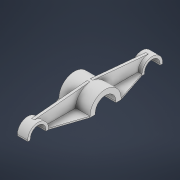
# Autodesk Inventor part: Pieza de practica 10
Saved by Autodesk Inventor 2022 (Build 260153000, 153)
## iProperties
Created: 2022-08-03
Part Number: Pieza de practica 10
Material: Genérico
Document SubType Name: Modeling
Designer: aleon
Density: 1 g/cm^3
Appearance: Valor por defecto
Author: aleon
Autodesk Inventor part; units mm, degrees
ref_plane "YZ Plane" through (0, 0, 0) normal (1, 0, 0) x (0, 1, 0)
ref_plane "XZ Plane" through (0, 0, 0) normal (0, 1, 0) x (-1, 0, 0)
ref_plane "XY Plane" through (0, 0, 0) normal (0, 0, 1) x (1, 0, 0)
sketch "Boceto1" plane through (0, 0, 0) normal (1, 0, 0) x (0, 1, 0)
  arc A0 (0, -20) -> (0, 20) centre (0, 0) ccw
  arc A1 (0, -30) -> (0, 30) centre (0, 0) ccw
  line L0 (0, 0) -> (-5, 0) construction
  arc A2 (0, -125) -> (0, -95) centre (0, -110) ccw
  arc A3 (0, -130) -> (0, -90) centre (0, -110) ccw
  arc A4 (0, 95) -> (0, 125) centre (0, 110) ccw
  arc A5 (0, 90) -> (0, 130) centre (0, 110) ccw
  line L1 (0, 95) -> (-2.5, 95)
  line L2 (-2.5, 95) -> (-2.5, 90)
  line L3 (-2.5, 90) -> (0, 90)
  line L4 (0, 125) -> (-2.5, 125)
  line L5 (-2.5, 125) -> (-2.5, 130)
  line L6 (-2.5, 130) -> (0, 130)
  line L7 (0, -95) -> (-2.5, -95)
  line L8 (-2.5, -95) -> (-2.5, -90)
  line L9 (-2.5, -90) -> (0, -90)
  line L10 (0, -125) -> (-2.5, -125)
  line L11 (-2.5, -125) -> (-2.5, -130)
  line L12 (-2.5, -130) -> (0, -130)
  line L13 (0, 20) -> (-2.5, 20)
  line L14 (-2.5, 20) -> (-2.5, 30)
  line L15 (-2.5, 30) -> (0, 30)
  line L16 (0, -20) -> (-2.5, -20)
  line L17 (-2.5, -20) -> (-2.5, -30)
  line L18 (-2.5, -30) -> (0, -30)
  point P0 (0, 130)
  dimension "d0" = 20
  dimension "d1" = 30
  dimension "d2" = 5
  dimension "d3" = 15
  dimension "d5" = 20
  dimension "d6" = 110
  dimension "d7" = 2.5
  dimension "d8" = 5
  dimension "d9" = 5
  dimension "d10" = 10
  dimension "d11" = 10
  dimension "d16" = 2.5
  constraints: 38 end point, 12 point on circle, 9 perpendicular, 6 centre point, 6 point on line, 6 symmetric about line, 4 coincident, 4 horizontal, 3 parallel, 2 other
  measures "d0" radius of A0
  measures "d1" radius of A1
  measures "d2" distance of L0.start L0.end
  measures "d3" radius of A2
  measures "d5" radius of A3
  measures "d6" distance of A2.centre point (0, 0)
  measures "d7" distance of L1.start L1.end
  measures "d8" distance of L7.end L8.end
  measures "d9" distance of L10.end L11.end
  measures "d10" distance of L13.end L14.end
  measures "d11" distance of L16.end L17.end
  measures "d16" distance of L8.end L9.end
extrude "Extrusión1" add sketch "Boceto1" along normal mid plane 60 contours A0 L13 L14 L15 A1 L18 L17 L16
extrude "Extrusión2" add sketch "Boceto1" along normal mid plane 20 contours A2 L7 L8 L9 A3 L12 L11 L10 | A4 L4 L5 L6 A5 L3 L2 L1
sketch "Boceto2" plane through (-30, -2.5, 20) normal (0, -1, 0) x (1, 0, 0)
  line L0 (40, 70) -> (20, 70) projected
  line L1 (40, 75) -> (40, 70) projected
  line L2 (60, 10) -> (40, 70)
  line L3 (0, 10) -> (60, 10) projected
  line L4 (20, 70) -> (0, 10)
  line L5 (60, -40) -> (60, -50) projected
  line L6 (60, -50) -> (40, -110)
  line L7 (20, -110) -> (0, -50)
  line L8 (0, -50) -> (60, -50) projected
  line L9 (60, -50) -> (0, -50)
  line L10 (60, 10) -> (60, 0) projected
  line L11 (60, 10) -> (0, 10)
  line L12 (20, -110) -> (40, -110) projected
  line L13 (40, -110) -> (20, -110)
  point P0 (30, -20)
  constraints: 15 end point, 2 horizontal, 1 perpendicular
extrude "Extrusión3" add sketch "Boceto2" against normal blind 2.5
sketch "Boceto3" plane through (0, 0, 0) normal (1, 0, 0) x (0, 1, 0)
  arc A0 (0, -130) -> (0, -90) centre (0, -110) ccw projected
  line L0 (20, -110) -> (29.8737, -2.7502)
  arc A1 (0, -30) -> (0, 30) centre (0, 0) ccw projected
  arc A2 (0, 90) -> (0, 130) centre (0, 110) ccw projected
  line L1 (20, 110) -> (29.9301, 2.1377)
  line L2 (0, -30) -> (0, -90) projected
  line L3 (0, 90) -> (0, 30) projected
  point P0 (29.8737, 2.7502)
  constraints: 4 end point, 3 point on circle, 2 tangent
extrude "Extrusión4" add sketch "Boceto3" along normal mid plane 5
